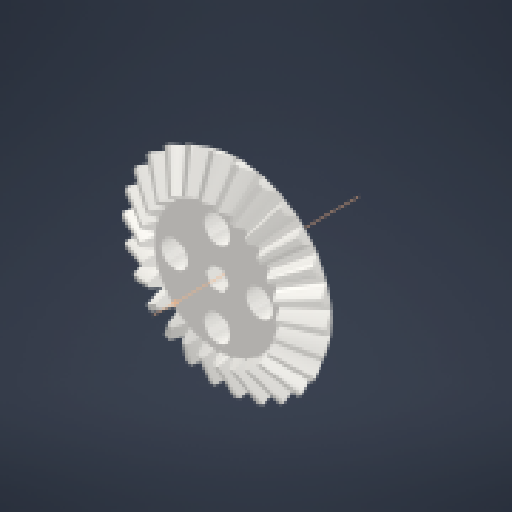
# Autodesk Inventor part: Bevel Gear1
Saved by Autodesk Inventor 2023 (Build 270158000, 158)
## iProperties
CustomPartVersion: 1
Created: 2022-11-09
Part Number: Bevel Gear1
Material: Steel, Mild
Document SubType Name: Modeling
Designer: izack
Categories: <?xml version="1.0" encoding="UTF-16"?> <MemberInstance><Categories><FamilyTemplate><FamilyTemplateParameter ValueType="xs:double" Id="1" ObjectReferenceKey="da_z" ObjectType="kUserParameterObject"/><FamilyTemplateParameter ValueType="xs:double" Id="2" ObjectReferenceKey="da_b" ObjectType="kUserParameterObject"/><FamilyTemplateParameter ValueType="xs:double" Id="3" ObjectReferenceKey="da_beta" ObjectType="kUserParameterObject"/><FamilyTemplateParameter ValueType="xs:double" Id="4" ObjectReferenceKey="da_dae" ObjectType="kUserParameterObject"/><FamilyTemplateParameter ValueType="xs:double" Id="5" ObjectReferenceKey="da_ve" ObjectType="kUserParameterObject"/><FamilyTemplateParameter ValueType="xs:double" Id="6" ObjectReferenceKey="da_omega" ObjectType="kUserParameterObject"/><FamilyTemplateParameter ValueType="xs:string" Id="7" ObjectReferenceKey="EAIAABAAAAAAHwAAAAAAAIAAAAAAAAAA" ObjectType="83914240" SubObjectId="SurfaceGeometry"/></FamilyTemplate><ParamToTemplateMap><ParamToTemplate CategoryParameter="//CategoryParameter[@InternalName='046C89C9-8512-4d59-83FE-43B91F4F132A']" TemplateParameter="1"/><ParamToTemplate CategoryParameter="//CategoryParameter[@InternalName='2552DF32-E462-4b46-AEBF-C6C7768E72AC']" TemplateParameter="2"/><ParamToTemplate CategoryParameter="//CategoryParameter[@InternalName='C9EE641D-15FC-4fae-A226-E94C4372FDD7']" TemplateParameter="3"/><ParamToTemplate><ParamToTemplate CategoryParameter="//CategoryParameter[@InternalName='00B6519A-459B-49c7-AD84-2E56D39A5744']" ConstantValue="0.000000"/></ParamToTemplate><ParamToTemplate><ParamToTemplate CategoryParameter="//CategoryParameter[@InternalName='04B31F0E-C7A6-4894-AA32-9629BEFACF47']" ConstantValue="1.000000"/></ParamToTemplate><ParamToTemplate><ParamToTemplate CategoryParameter="//CategoryParameter[@InternalName='43CBEC2E-7847-49e7-A936-2F7889FCB2D9']" ConstantValue="0.200000"/></ParamToTemplate><ParamToTemplate><ParamToTemplate CategoryParameter="//CategoryParameter[@InternalName='B1EFC894-105D-4ebd-86BF-FA20ED196853']" ConstantValue="0.300000"/></ParamToTemplate><ParamToTemplate><ParamToTemplate CategoryParameter="//CategoryParameter[@InternalName='51175063-3D10-4879-93E8-6246FE8B403D']" ConstantValue="2060000000.000000"/></ParamToTemplate><ParamToTemplate><ParamToTemplate CategoryParameter="//CategoryParameter[@InternalName='A3A52E27-4454-46a9-B0BD-C932399B70AF']" ConstantValue="0.300000"/></ParamToTemplate><ParamToTemplate CategoryParameter="//CategoryParameter[@InternalName='2A200944-5A8C-41ca-B96E-8520D2E510F1']" TemplateParameter="4"/><ParamToTemplate><ParamToTemplate CategoryParameter="//CategoryParameter[@InternalName='1A637F62-92C8-44bc-B81F-10802510B579']" ConstantValue="3.600925"/></ParamToTemplate><ParamToTemplate CategoryParameter="//CategoryParameter[@InternalName='B52DD4BE-6863-48fb-BF58-89EF6F9EC65C']" TemplateParameter="5"/><ParamToTemplate><ParamToTemplate CategoryParameter="//CategoryParameter[@InternalName='3956BFF2-84D2-457d-93C2-9B0613DEBA67']" ConstantValue="0.884754"/></ParamToTemplate><ParamToTemplate CategoryParameter="//CategoryParameter[@InternalName='739CFA02-461B-4bf8-8049-181FCAD8B28F']" TemplateParameter="6"/><ParamToTemplate><ParamToTemplate CategoryParameter="//CategoryParameter[@InternalName='A27E999F-E2CE-4481-8A2A-EBF499C4C3C5']" ConstantValue="0.000000"/></ParamToTemplate><ParamToTemplate><ParamToTemplate CategoryParameter="//CategoryParameter[@InternalName='9E1B4470-B2D3-4ff1-B813-535BB4CDF51A']" ConstantValue="3520000.000000"/></ParamToTemplate><ParamToTemplate><ParamToTemplate CategoryParameter="//CategoryParameter[@InternalName='F8452263-BFF6-458c-9FB1-07C4B99E95CD']" ConstantValue="11400000.000000"/></ParamToTemplate><ParamToTemplate><ParamToTemplate CategoryParameter="//CategoryParameter[@InternalName='3E3BB259-FD49-497f-8171-6EBC954A3479']" ConstantValue="2.000000"/></ParamToTemplate><ParamToTemplate CategoryParameter="//CategoryParameter[@InternalName='27C3BAF2-7550-4e4b-AE2C-0DB134B7D9B7']" TemplateParameter="7"/></ParamToTemplateMap><Category DisplayName="Gear" InternalName="DC85795E-93AB-48d5-8EEE-5A27447B64BD" Mnemonic="Gear"><CategoryParameter DisplayName="z" InternalName="046C89C9-8512-4d59-83FE-43B91F4F132A" Mnemonic="z"/><CategoryParameter DisplayName="b" InternalName="2552DF32-E462-4b46-AEBF-C6C7768E72AC" Mnemonic="b"/><CategoryParameter DisplayName="||b|" InternalName="C9EE641D-15FC-4fae-A226-E94C4372FDD7" Mnemonic="beta"/><CategoryParameter DisplayName="x" InternalName="00B6519A-459B-49c7-AD84-2E56D39A5744" Mnemonic="x"/><CategoryParameter DisplayName="a*" InternalName="04B31F0E-C7A6-4894-AA32-9629BEFACF47" Mnemonic="a"/><CategoryParameter DisplayName="c*" InternalName="43CBEC2E-7847-49e7-A936-2F7889FCB2D9" Mnemonic="c"/><CategoryParameter DisplayName="r|.f|*" InternalName="B1EFC894-105D-4ebd-86BF-FA20ED196853" Mnemonic="rf"/><CategoryParameter DisplayName="E" InternalName="51175063-3D10-4879-93E8-6246FE8B403D" Mnemonic="E"/><CategoryParameter DisplayName="||m|" InternalName="A3A52E27-4454-46a9-B0BD-C932399B70AF" Mnemonic="mi"/><Category DisplayName="BevelGear" InternalName="0C98F69A-0C2B-4791-B2FE-7691BB227E77" Mnemonic="BevelGear"><CategoryParameter DisplayName="d|.ae|" InternalName="2A200944-5A8C-41ca-B96E-8520D2E510F1" Mnemonic="dae"/><CategoryParameter DisplayName="d|.ai|" InternalName="1A637F62-92C8-44bc-B81F-10802510B579" Mnemonic="dai"/><CategoryParameter DisplayName="A|.e|" InternalName="B52DD4BE-6863-48fb-BF58-89EF6F9EC65C" Mnemonic="ve"/><CategoryParameter DisplayName="A|.i|" InternalName="3956BFF2-84D2-457d-93C2-9B0613DEBA67" Mnemonic="vi"/><CategoryParameter DisplayName="||S|" InternalName="739CFA02-461B-4bf8-8049-181FCAD8B28F" Mnemonic="omega"/><CategoryParameter DisplayName="x|.t|" InternalName="A27E999F-E2CE-4481-8A2A-EBF499C4C3C5" Mnemonic="xt"/><CategoryParameter DisplayName="||s||.Flim|" InternalName="9E1B4470-B2D3-4ff1-B813-535BB4CDF51A" Mnemonic="sFlim"/><CategoryParameter DisplayName="||s||.Hlim|" InternalName="F8452263-BFF6-458c-9FB1-07C4B99E95CD" Mnemonic="sHlim"/><CategoryParameter DisplayName="type" InternalName="3E3BB259-FD49-497f-8171-6EBC954A3479" Mnemonic="type"/><CategoryParameter DisplayName="PitchDiameter" InternalName="27C3BAF2-7550-4e4b-AE2C-0DB134B7D9B7" Mnemonic="IDS_PITCHDIAM"/></Category></Category></Categories></MemberInstance>
Mass: 60.9118 g
Surface Area: 34.3074 cm^2
Volume: 7.7496 cm^3
Density: 7.86 g/cm^3
Appearance: Steel
Author: izack
## iProperties of the stored document Bevel Gear11_3DPrint.ipt
Part Number: Bevel Gear11_3DPrint
Material: Generic
Document SubType Name: Modeling
Designer: izack
Appearance: Default
Author: izack
Autodesk Inventor part; units mm, degrees
ref_plane "Mesh Plane2" through (0, 0, 0) normal (0.9927089, 0.1205367, 0) x (0, 0, 1)
sketch "Teeth Body Sketch" plane through (0, 0, 0) normal (1, 0, 0) x (0, 1, 0)
  line L0 (0, 0) -> (24.800666, -17.078845) construction
  line L1 (24.800666, -17.078845) -> (26.999445, -13.267629)
  line L2 (26.999445, -13.267629) -> (0, 0) construction
  line L3 (26, -15) -> (0, 0) construction
  line L4 (16.538366, -11.389057) -> (18.004626, -8.847541)
  line L5 (24.800666, -17.078845) -> (16.538366, -11.389057)
  line L6 (26.999445, -13.267629) -> (18.004626, -8.847541)
  line L7 (0, -20.198363) -> (0, 3.366394)
  line L8 (0, -15) -> (26.999445, -15) construction
  dimension "d0" = 52
  dimension "d1" = 49.60133
  dimension "d2" = 53.99889
  dimension "d3" = 10
  dimension "d4" = 13.26763
  constraints: 16 end point, 4 point on line, 3 perpendicular, 2 collinear, 1 horizontal alignment, 1 vertical alignment
  measures "d0" diameter of L3.start L7
  measures "d1" diameter of L0.end L7
  measures "d2" diameter of L1.end L7
  measures "d3" distance between parallel lines of L1 L4
  measures "d4" vertical distance of L1.end L0.start
revolve "Teeth Body" add sketch "Teeth Body Sketch" angle 360 about axis through (0, 0, 0) along (0, 0, 1)
ref_plane "Tooth Plane" through (0, 26, -15) normal (0, -0.8661856, 0.4997225) x (1, 0, 0)
sketch "Start Sketch" plane through (0, 26, -15) normal (0, -0.8661856, 0.4997225) x (1, 0, 0)
  line L0 (0, -105.588298) -> (0, 23.440092)
  arc A0 (-0.713811, -2.927999) -> (-3.252253, 3.224369) centre (-18.791416, -6.786886) ccw
  arc A1 (3.252253, 3.224369) -> (0.713811, -2.927999) centre (18.791416, -6.786886) ccw
  line L1 (-0.713811, -2.927999) -> (0.713811, -2.927999)
  arc A2 (3.252253, 3.224369) -> (-3.252253, 3.224369) centre (0, -52.02888) ccw
  dimension "d7" = 18.48488
  dimension "d8" = 18.79142
  dimension "d9" = 45.24199
  dimension "d57" = 55.34888
  dimension "d58" = 49.10088
  constraints: 6 point on circle, 3 centre point, 3 symmetric about line, 2 end point, 1 coincident, 1 perpendicular, 1 other
  measures "d7" radius of A0
  measures "d8" horizontal distance of point (0, -52.029) A0.centre
  measures "d9" vertical distance of point (0, -52.029) A0.centre
  measures "d57" radius of A2
  measures "d58" distance from line of A2.centre L1
sketch "End Sketch" plane through (0, 17.147583, -9.892837) normal (0, -0.8661856, 0.4997225) x (1, 0, 0)
  line L0 (0, -80.919653) -> (0, 17.963771)
  arc A0 (-0.470774, -1.931082) -> (-2.144934, 2.126543) centre (-12.393361, -4.476104) ccw
  arc A1 (2.144934, 2.126543) -> (0.470774, -1.931082) centre (12.393361, -4.476104) ccw
  line L1 (-0.470774, -1.931082) -> (0.470774, -1.931082)
  arc A2 (2.144934, 2.126543) -> (-2.144934, 2.126543) centre (0, -34.314214) ccw
  dimension "d12" = 12.19119
  dimension "d15" = 12.39336
  dimension "d16" = 29.83811
  dimension "d59" = 36.50383
  dimension "d60" = 32.38313
  constraints: 6 point on circle, 3 centre point, 3 symmetric about line, 2 end point, 1 coincident, 1 other
  measures "d12" radius of A0
  measures "d15" horizontal distance of A0.centre point (0, -34.314)
  measures "d16" vertical distance of A0.centre point (0, -34.314)
  measures "d59" radius of A2
  measures "d60" distance from line of A2.centre L1
loft "Loft" cut profiles "Start Sketch", "End Sketch"
pattern_circular "Circular Pattern" count 26 over 360 about axis through (0, 0, 0) along (0, 0, 1) of "Loft"
ref_plane "End Plane" through (0, 17.147583, -9.892837) normal (0, -0.8661856, 0.4997225) x (1, 0, 0)
sketch3d "3D Sketch Right"
ref_plane "End Plane Right" through (-2.316557, 16.990385, -9.892837) normal (0.1170175, -0.8582449, 0.4997225) x (0.9908326, 0.1350952, 0)
sketch "End Sketch Right" plane through (-2.316557, 16.990385, -9.892837) normal (0.1170175, -0.8582449, 0.4997225) x (0.9908326, 0.1350952, 0)
  arc A0 (-0.470774, -1.931082) -> (-2.144934, 2.126543) centre (-12.393361, -4.476104) ccw
  line L0 (0, -85.389338) -> (0, 22.433456)
  arc A1 (2.144934, 2.126543) -> (0.470774, -1.931082) centre (12.393361, -4.476104) ccw
  line L1 (-0.470774, -1.931082) -> (0.470774, -1.931082)
  arc A2 (2.144934, 2.126543) -> (-2.144934, 2.126543) centre (0, -34.314214) ccw
  dimension "d70" = 12.39336
  dimension "d71" = 29.83811
  dimension "d72" = 12.19119
  dimension "d73" = 32.38313
  dimension "d74" = 36.50383
  constraints: 6 point on circle, 3 centre point, 3 symmetric about line, 2 end point, 1 coincident, 1 perpendicular, 1 other
  measures "d70" horizontal distance of A2.centre A0.centre
  measures "d71" vertical distance of point (0, -34.314) A0.centre
  measures "d72" radius of A0
  measures "d73" distance from line of point (0, -34.314) L1
  measures "d74" radius of A2
feature "Loft Right" [suppressed]
pattern_circular "Circular Pattern Right" [suppressed]
sketch3d "3D Sketch Left"
ref_plane "End Plane Left" through (2.316062, 16.990385, -9.892612) normal (-0.1169935, -0.8582523, 0.4997154) x (0.9908365, -0.1350669, 0)
sketch "End Sketch Left" plane through (2.316062, 16.990385, -9.892612) normal (-0.1169935, -0.8582523, 0.4997154) x (0.9908365, -0.1350669, 0)
  line L0 (0, -85.855634) -> (0, 22.943521)
  arc A0 (-0.470774, -1.931243) -> (-2.144934, 2.126382) centre (-12.393361, -4.476265) ccw
  arc A1 (2.144934, 2.126382) -> (0.470774, -1.931243) centre (12.393361, -4.476265) ccw
  line L1 (-0.470774, -1.931243) -> (0.470774, -1.931243)
  ellipse E0 centre (0, -7.663648) end of major axis (18.004626, -7.663648) minor radius 8.997189
  arc A2 (2.144934, 2.126382) -> (-2.144934, 2.126382) centre (0, -34.314375) ccw
  dimension "d56" = 8.99719
  dimension "d30" = 12.19119
  dimension "d31" = 12.39336
  dimension "d32" = 29.83811
  dimension "d61" = 36.50383
  dimension "d62" = 32.38313
  constraints: 6 point on circle, 3 centre point, 3 symmetric about line, 2 end point, 1 coincident, 2 other
  measures "d30" radius of A0
  measures "d31" horizontal distance of point (0, -34.314) A0.centre
  measures "d32" vertical distance of A0.centre point (0, -34.314)
  measures "d61" radius of A2
  measures "d62" distance from line of point (0, -34.314) L1
feature "Loft Left" [suppressed]
pattern_circular "Circular Pattern Left" [suppressed]
sketch "Body Sketch" plane through (0, 0, 0) normal (1, 0, 0) x (0, 1, 0)
  line L0 (0, -17.587304) -> (0, -12.299961)
  line L1 (24.800666, -17.078845) -> (16.538366, -11.389057)
  line L2 (16.538366, -11.389057) -> (0, -11.389057)
  line L3 (24.800666, -17.078845) -> (0, -17.078845)
  constraints: 4 end point, 2 perpendicular, 2 point on line
sketch "Body Sketch outline for Fix Body" plane through (0, 0, 0) normal (1, 0, 0) x (0, 1, 0)
  line L0 (0, -17.078845) -> (24.800666, -17.078845)
  line L1 (0, -11.389057) -> (0, -17.078845)
  line L2 (16.538366, -11.389057) -> (0, -11.389057)
  line L3 (24.800666, -17.078845) -> (16.538366, -11.389057)
revolve "Fix Body" add sketch "Body Sketch outline for Fix Body" angle 360 about axis through (0, 0, 0) along (0, 0, 1)
sketch "Sketch6" plane through (0, 0, 0) normal (1, 0, 0) x (0, 1, 0)
  line L0 (26, -15) -> (0, 0) projected
  line L1 (0, -16.2) -> (0, 2.7) projected
surface revolve "Pitch Diameter" sketch "Sketch6" angle 360 about axis through (0, 0, 0) along (0, 0, 1) shown no curves L0
sketch "Sketch8" plane through (0, 0, -11.389057) normal (0, 0, 1) x (1, 0, 0)
  circle A0 centre (0, 0) radius 2.65
  line L0 (-1.529978, -2.65) -> (-3.059956, 0)
  line L1 (-3.059956, 0) -> (-1.529978, 2.65)
  line L2 (-1.529978, 2.65) -> (1.529978, 2.65)
  line L3 (1.529978, 2.65) -> (3.059956, 0)
  line L4 (3.059956, 0) -> (1.529978, -2.65)
  line L5 (1.529978, -2.65) -> (-1.529978, -2.65)
  circle A1 centre (0, 0) radius 6
  circle A2 centre (0, 0) radius 11.34 construction
  circle A3 centre (0, -11.34) radius 3.5
  circle A4 centre (11.34, 0) radius 3.5
  circle A5 centre (0, 11.34) radius 3.5
  circle A6 centre (-11.34, 0) radius 3.5
  point P0 (0, -2.65)
  point P1 (-5.484375, 2.43344)
  point P2 (-5.484375, -2.43344)
  point P3 (-2.43344, -5.484375)
  point P4 (2.43344, -5.484375)
  point P5 (5.484375, -2.43344)
  point P6 (5.484375, 2.43344)
  point P7 (2.43344, 5.484375)
  point P8 (-2.43344, 5.484375)
  dimension "d94" = 5.3
  dimension "d100" = 22.68
  dimension "d95" = 12
  dimension "d101" = 7
  dimension "d104" = 360
  constraints: 12 end point, 5 centre point, 4 coincident, 2 vertical alignment, 1 midpoint, 26 other
  measures "d95" diameter of A1
  measures "d101" diameter of A3
extrude "Extrusion1" cut sketch "Sketch8" against normal through all contours A0 | A0 L3 L4 | A0 L2 L3 | L4 L5 A0 | A0 L1 L2 | L5 L0 A0 | A0 L0 L1 | A3 | A4 | A5 | A6
ref_plane "Work Plane6" through (-11.017772, -11.017772, -23.9) normal (0, 0, 1) x (0.9370518, 0.3491903, 0)
extrude "Extrusion2" add sketch "Sketch8" against normal up to surface (12.510943 mm away) contours A1
equation "\"d0\" = da_de"
equation "\"d1\" = da_dfe"
equation "\"d2\" = da_dae"
equation "\"d3\" = da_b"
equation "\"d4\" = da_ve"
equation "\"d7\" = fd_rr"
equation "\"d8\" = fd_x"
equation "\"d9\" = fd_y"
equation "\"d57\" = 0.5 * fd_dva + 0.3 * da_he"
equation "\"d58\" = 0.5 * fd_dva - 1.12 * da_he"
equation "\"da_teethtype\" = 0"
equation "\"da_b\" = 10"
equation "\"da_de\" = 52"
equation "\"da_dae\" = 53.99889"
equation "\"da_dfe\" = 49.60133"
equation "\"da_le\" = 30.01666"
equation "\"da_omega\" = 90deg"
equation "\"da_beta\" = 0"
equation "\"da_delta\" = 60.018361deg"
equation "\"da_alpha\" = 20deg"
equation "\"da_he\" = 4.4"
equation "\"da_ve\" = 13.26763"
equation "\"da_zv\" = 52.028881"
equation "\"fd_loft\" = da_b + 0.05 * da_he"
equation "\"fd_x\" = fd_x1 + fd_x2"
equation "\"fd_y\" = fd_y1 - fd_y2"
equation "\"fd_dd\" = fd_dva - 0.8 * da_he"
equation "\"da_dvw\" = 104.05776"
equation "\"d11\" = fd_loft"
equation "\"da_dm\" = 43.33814"
equation "\"da_x\" = 0"
equation "\"da_m\" = 2"
equation "\"d50\" = da_omega"
equation "\"fd_rr\" = 18.484881"
equation "\"fd_dva\" = 108.057762"
equation "\"fd_x1\" = 1.588003"
equation "\"fd_x2\" = 17.203413"
equation "\"fd_y1\" = 52.004641"
equation "\"fd_y2\" = 6.762647"
body "Solid1"
body "Srf1"
